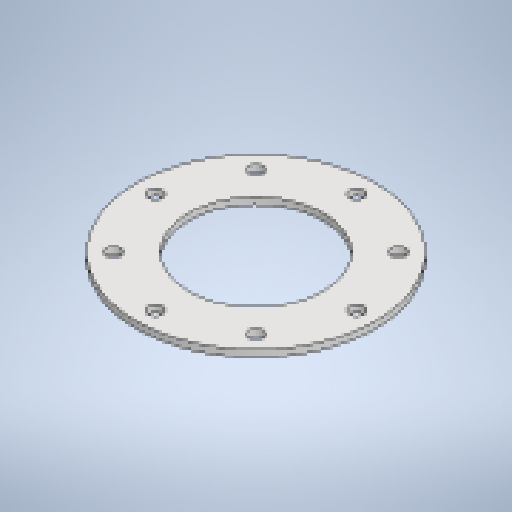
# Autodesk Inventor part: PNS 1706 charging flange round
Saved by Autodesk Inventor 2025.1 (Build 291241020, 241B)
## iProperties
Created: 2025-02-13
Part Number: PNS 1706 charging flange round
Material: Steel
Document SubType Name: Sheet Metal
Designer: admin
Density: 7.85 g/cm^3
Sheet Metal Rule: AISI304 4mm Die 32
Sheet Metal Width: 285.000 mm
Sheet Metal Length: 285.000 mm
Sheet Metal Area: 81225.000 mm^2
Appearance: Default
Mass: 2466.79 g
Surface Area: 934.137 cm^2
Volume: 314.241 cm^3
Flat Pattern Width: 28.5 cm
Flat Pattern Length: 28.5 cm
Flat Pattern Area: 812.25 cm^2
Author: pokla
Autodesk Inventor part; units mm, degrees
ref_plane "YZ Plane" through (0, 0, 0) normal (1, 0, 0) x (0, 1, 0)
ref_plane "XZ Plane" through (0, 0, 0) normal (0, 1, 0) x (-1, 0, 0)
ref_plane "XY Plane" through (0, 0, 0) normal (0, 0, 1) x (1, 0, 0)
sketch "Sketch2" plane through (0, 0, 0) normal (0, 0, 1) x (1, 0, 0)
  circle A0 centre (0, 0) radius 80.5
  circle A1 centre (0, 0) radius 142.5
  dimension "d25" = 161
  dimension "d27" = 285
  measures "d25" diameter of A0
  measures "d27" diameter of A1
extrude "Plate2" add sketch "Sketch2" along normal blind 8
sketch "Sketch3" plane through (0, 0, 8) normal (0, 0, 1) x (1, 0, 0)
  circle A0 centre (-120, 0) radius 8.5
  circle A1 centre (0, 0) radius 120 construction
  dimension "d28" = 240
  dimension "d15" = 17
  constraints: 2 horizontal alignment, 1 centre point, 1 coincident, 2 other
  measures "d15" diameter of A0
extrude "Cut1" cut sketch "Sketch3" against normal blind 8
pattern_circular "Circular Pattern1" count 8 over 360 about axis through (0, 0, 0) along (0, 0, 1) of "Cut1"
equation "\"d17\" = Thickness"
equation "\"d14\" = Thickness"
equation "\"BendReliefWidth\" = Thickness"
equation "\"BendReliefDepth\" = 0.5 * Thickness"
equation "\"CornerReliefSize\" = 4 * Thickness"
equation "\"MinimumRemnant\" = 2 * Thickness"
equation "\"TransitionRadius\" = BendRadius"
equation "\"JacobiRadiusSize\" = BendRadius"
equation "\"GapSize\" = Thickness"
equation "\"Thickness\" = 8"
equation "\"BendRadius\" = 6"
body "Solid3"
